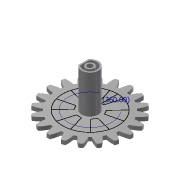
# Autodesk Inventor part: Spur Gear2
Saved by Autodesk Inventor 2018 (Build 220112000, 112)
## iProperties
Created: 2018-10-24
Part Number: Spur Gear2
Material: Steel
Document SubType Name: Modeling
Designer: Vulnic
Categories: <?xml version="1.0" encoding="UTF-16"?> <MemberInstance><Categories><FamilyTemplate><FamilyTemplateParameter ValueType="xs:double" Id="1" ObjectReferenceKey="da_z" ObjectType="kUserParameterObject"/><FamilyTemplateParameter ValueType="xs:double" Id="2" ObjectReferenceKey="da_b" ObjectType="kUserParameterObject"/><FamilyTemplateParameter ValueType="xs:double" Id="3" ObjectReferenceKey="da_beta" ObjectType="kUserParameterObject"/><FamilyTemplateParameter ValueType="xs:double" Id="4" ObjectReferenceKey="da_da" ObjectType="kUserParameterObject"/><FamilyTemplateParameter ValueType="xs:double" Id="5" ObjectReferenceKey="da_aw" ObjectType="kUserParameterObject"/><FamilyTemplateParameter ValueType="xs:string" Id="6" ObjectReferenceKey="EAIAABAAAACIAQAAAAAAAIAAAAAAAAAA" ObjectType="83910656" SubObjectId="SurfaceGeometry"/></FamilyTemplate><ParamToTemplateMap><ParamToTemplate CategoryParameter="//CategoryParameter[@InternalName='046C89C9-8512-4d59-83FE-43B91F4F132A']" TemplateParameter="1"/><ParamToTemplate CategoryParameter="//CategoryParameter[@InternalName='2552DF32-E462-4b46-AEBF-C6C7768E72AC']" TemplateParameter="2"/><ParamToTemplate CategoryParameter="//CategoryParameter[@InternalName='C9EE641D-15FC-4fae-A226-E94C4372FDD7']" TemplateParameter="3"/><ParamToTemplate><ParamToTemplate CategoryParameter="//CategoryParameter[@InternalName='00B6519A-459B-49c7-AD84-2E56D39A5744']" ConstantValue="0.000000"/></ParamToTemplate><ParamToTemplate><ParamToTemplate CategoryParameter="//CategoryParameter[@InternalName='04B31F0E-C7A6-4894-AA32-9629BEFACF47']" ConstantValue="1.000000"/></ParamToTemplate><ParamToTemplate><ParamToTemplate CategoryParameter="//CategoryParameter[@InternalName='43CBEC2E-7847-49e7-A936-2F7889FCB2D9']" ConstantValue="0.250000"/></ParamToTemplate><ParamToTemplate><ParamToTemplate CategoryParameter="//CategoryParameter[@InternalName='B1EFC894-105D-4ebd-86BF-FA20ED196853']" ConstantValue="0.350000"/></ParamToTemplate><ParamToTemplate><ParamToTemplate CategoryParameter="//CategoryParameter[@InternalName='51175063-3D10-4879-93E8-6246FE8B403D']" ConstantValue="2060000000.000000"/></ParamToTemplate><ParamToTemplate><ParamToTemplate CategoryParameter="//CategoryParameter[@InternalName='A3A52E27-4454-46a9-B0BD-C932399B70AF']" ConstantValue="0.300000"/></ParamToTemplate><ParamToTemplate><ParamToTemplate CategoryParameter="//CategoryParameter[@InternalName='91B76062-C214-41d9-B1B9-14D2AB99603D']" ConstantValue="0.100000"/></ParamToTemplate><ParamToTemplate><ParamToTemplate CategoryParameter="//CategoryParameter[@InternalName='374E806E-8B8A-4dda-A9AA-1039D6500AD2']" ConstantValue="10.000000"/></ParamToTemplate><ParamToTemplate><ParamToTemplate CategoryParameter="//CategoryParameter[@InternalName='2D373A89-B862-43d6-8D0B-0CBF12AB9F6C']" ConstantValue="0.349066"/></ParamToTemplate><ParamToTemplate CategoryParameter="//CategoryParameter[@InternalName='37777632-D6A2-4fac-9D53-DB8ACD95C989']" TemplateParameter="4"/><ParamToTemplate CategoryParameter="//CategoryParameter[@InternalName='FD1017F1-B727-4f7e-9707-0F86F1FF9423']" TemplateParameter="5"/><ParamToTemplate><ParamToTemplate CategoryParameter="//CategoryParameter[@InternalName='9E1B4470-B2D3-4ff1-B813-535BB4CDF51A']" ConstantValue="3520000.000000"/></ParamToTemplate><ParamToTemplate><ParamToTemplate CategoryParameter="//CategoryParameter[@InternalName='F8452263-BFF6-458c-9FB1-07C4B99E95CD']" ConstantValue="11400000.000000"/></ParamToTemplate><ParamToTemplate><ParamToTemplate CategoryParameter="//CategoryParameter[@InternalName='3E3BB259-FD49-497f-8171-6EBC954A3479']" ConstantValue="2.000000"/></ParamToTemplate><ParamToTemplate CategoryParameter="//CategoryParameter[@InternalName='27C3BAF2-7550-4e4b-AE2C-0DB134B7D9B7']" TemplateParameter="6"/></ParamToTemplateMap><Category DisplayName="Gear" InternalName="DC85795E-93AB-48d5-8EEE-5A27447B64BD" Mnemonic="Gear"><CategoryParameter DisplayName="z" InternalName="046C89C9-8512-4d59-83FE-43B91F4F132A" Mnemonic="z"/><CategoryParameter DisplayName="b" InternalName="2552DF32-E462-4b46-AEBF-C6C7768E72AC" Mnemonic="b"/><CategoryParameter DisplayName="||b|" InternalName="C9EE641D-15FC-4fae-A226-E94C4372FDD7" Mnemonic="beta"/><CategoryParameter DisplayName="x" InternalName="00B6519A-459B-49c7-AD84-2E56D39A5744" Mnemonic="x"/><CategoryParameter DisplayName="a*" InternalName="04B31F0E-C7A6-4894-AA32-9629BEFACF47" Mnemonic="a"/><CategoryParameter DisplayName="c*" InternalName="43CBEC2E-7847-49e7-A936-2F7889FCB2D9" Mnemonic="c"/><CategoryParameter DisplayName="r|.f|*" InternalName="B1EFC894-105D-4ebd-86BF-FA20ED196853" Mnemonic="rf"/><CategoryParameter DisplayName="E" InternalName="51175063-3D10-4879-93E8-6246FE8B403D" Mnemonic="E"/><CategoryParameter DisplayName="||m|" InternalName="A3A52E27-4454-46a9-B0BD-C932399B70AF" Mnemonic="mi"/><Category DisplayName="SpurGear" InternalName="26C5A22E-A91E-4dfd-A3B3-23CCAFAE1764" Mnemonic="SpurGear"><CategoryParameter DisplayName="m" InternalName="91B76062-C214-41d9-B1B9-14D2AB99603D" Mnemonic="m"/><CategoryParameter DisplayName="P" InternalName="374E806E-8B8A-4dda-A9AA-1039D6500AD2" Mnemonic="PP"/><CategoryParameter DisplayName="||a|" InternalName="2D373A89-B862-43d6-8D0B-0CBF12AB9F6C" Mnemonic="alpha"/><CategoryParameter DisplayName="d|.a|" InternalName="37777632-D6A2-4fac-9D53-DB8ACD95C989" Mnemonic="da"/><CategoryParameter DisplayName="a|.w|" InternalName="FD1017F1-B727-4f7e-9707-0F86F1FF9423" Mnemonic="aw"/><CategoryParameter DisplayName="||s||.Flim|" InternalName="9E1B4470-B2D3-4ff1-B813-535BB4CDF51A" Mnemonic="sFlim"/><CategoryParameter DisplayName="||s||.Hlim|" InternalName="F8452263-BFF6-458c-9FB1-07C4B99E95CD" Mnemonic="sHlim"/><CategoryParameter DisplayName="type" InternalName="3E3BB259-FD49-497f-8171-6EBC954A3479" Mnemonic="type"/><CategoryParameter DisplayName="PitchDiameter" InternalName="27C3BAF2-7550-4e4b-AE2C-0DB134B7D9B7" Mnemonic="IDS_PITCHDIAM"/></Category></Category></Categories></MemberInstance>
Density: 1 g/cm^3
Appearance: Steel
CustomPartVersion: 1
Author: Vulnic
Autodesk Inventor part; units mm, degrees
ref_plane "YZ Plane" through (0, 0, 0) normal (1, 0, 0) x (0, 1, 0)
ref_plane "XZ Plane" through (0, 0, 0) normal (0, 1, 0) x (-1, 0, 0)
ref_plane "XY Plane" through (0, 0, 0) normal (0, 0, 1) x (1, 0, 0)
sketch "Sketch1" plane through (0, 0, 0) normal (0, 0, 1) x (1, 0, 0)
  circle A0 centre (0, 0) radius 11
  dimension "d0" = 22
  constraints: 1 centre point
  measures "d0" diameter of A0
extrude "Extrusion1" add sketch "Sketch1" along normal blind 1
ref_plane "Work Plane2" through (0, 0, 0.5) normal (0, 0, 1) x (1, 0, 0)
sketch "Sketch2" plane through (0, 0, 0) normal (0, 0, -1) x (-1, 0, 0)
  circle A0 centre (0, 0) radius 11 projected
  circle A1 centre (0, 0) radius 10
  dimension "d3" = 20
  constraints: 1 centre point, 1 coincident
  measures "d3" diameter of A1
surface extrude "Pitch Diameter" sketch "Sketch2" against normal through all shown no curves A1
ref_plane "Work Plane8" through (0, 0, 0) normal (0.9876883, 0.1564345, 0) x (0, 0, 1)
ref_plane "Work Plane9" through (0, 0, 0) normal (1, 0, 0) x (0, 1, 0)
spur gear teeth "Spur Gear" teeth 20 pitch diameter 20 tip diameter 22 root diameter 17.5 face width 1 start plane through (0, 0, 0) normal (0, 0, -1) x (-1, 0, 0)
sketch "Sketch3" plane through (0, 0, 1) normal (0, 0, 1) x (1, 0, 0)
  circle A0 centre (0, 0) radius 2.2 projected
  line L0 (-1.7577, -1.323) -> (-1.7577, 1.323)
  point P0 (0, 0)
  dimension "d49" = 2.646
  constraints: 2 end point, 2 point on circle, 1 vertical
  measures "d49" distance of L0.start L0.end
extrude "Extrusion2" cut sketch "Sketch3" against normal through all contours A0 L0 picked at (-0.4385, 0)
sketch "Sketch4" plane through (0, 0, 1) normal (0, 0, 1) x (1, 0, 0)
  line L0 (-0.6517, 2.9374) -> (0.0047, 2.9374)
  line L1 (0.0047, 2.9374) -> (0.0047, 7.2274)
  circle A0 centre (0, 0) radius 7.2274
  line L2 (-0.6517, 2.9374) -> (-1.8312, 6.9916)
  line L3 (0.6611, 2.9374) -> (0.0047, 2.9374)
  line L4 (0.6611, 2.9374) -> (1.8406, 6.9916)
  line L5 (-2.2133, 2.0412) -> (-5.1346, 5.0898)
  line L6 (-2.2133, 2.0412) -> (-2.5415, 1.4727)
  line L7 (-2.8697, 0.9043) -> (-2.5415, 1.4727)
  line L8 (-2.8697, 0.9043) -> (-6.9705, 1.91)
  line L9 (-2.8744, -0.8961) -> (-6.9752, -1.9018)
  line L10 (-2.8744, -0.8961) -> (-2.5462, -1.4646)
  line L11 (-2.218, -2.0331) -> (-2.5462, -1.4646)
  line L12 (-2.218, -2.0331) -> (-5.1393, -5.0817)
  line L13 (-0.6611, -2.9374) -> (-1.8406, -6.9916)
  line L14 (-0.6611, -2.9374) -> (-0.0047, -2.9374)
  line L15 (0.6517, -2.9374) -> (-0.0047, -2.9374)
  line L16 (0.6517, -2.9374) -> (1.8312, -6.9916)
  line L17 (2.2133, -2.0412) -> (5.1346, -5.0898)
  line L18 (2.2133, -2.0412) -> (2.5415, -1.4727)
  line L19 (2.8697, -0.9043) -> (2.5415, -1.4727)
  line L20 (2.8697, -0.9043) -> (6.9705, -1.91)
  line L21 (2.8744, 0.8961) -> (6.9752, 1.9018)
  line L22 (2.8744, 0.8961) -> (2.5462, 1.4646)
  line L23 (2.218, 2.0331) -> (2.5462, 1.4646)
  line L24 (2.218, 2.0331) -> (5.1393, 5.0817)
  line L25 (0.6611, 2.9374) -> (0.0047, 2.9374)
  line L26 (0.6611, 2.9374) -> (1.8406, 6.9916)
  line L27 (2.8744, 0.8961) -> (2.218, 2.0331)
  line L28 (5.1393, 5.0817) -> (2.218, 2.0331)
  line L29 (2.8744, 0.8961) -> (7.0083, 1.91)
  line L30 (6.9705, -1.91) -> (2.9023, -0.9123)
  line L31 (2.2133, -2.0412) -> (5.133, -5.0881)
  line L32 (1.8312, -6.9916) -> (0.6517, -2.9374)
  line L33 (-0.6611, -2.9374) -> (0.6517, -2.9374)
  line L34 (-0.6611, -2.9374) -> (-1.8406, -6.9916)
  line L35 (2.2133, -2.0412) -> (2.8697, -0.9043)
  line L36 (2.2133, -2.0412) -> (5.133, -5.0881)
  line L37 (-2.218, -2.0331) -> (-2.8744, -0.8961)
  line L38 (-2.8744, -0.8961) -> (-6.9752, -1.9018)
  line L39 (-5.1393, -5.0817) -> (-2.218, -2.0331)
  line L40 (-6.9705, 1.91) -> (-2.8697, 0.9043)
  line L41 (-2.8697, 0.9043) -> (-2.2133, 2.0412)
  line L42 (-2.2133, 2.0412) -> (-5.1346, 5.0898)
  arc A1 (-6.9705, -1.91) -> (-5.1393, -5.0817) centre (0, 0) ccw
  dimension "d54" = 360
  constraints: 86 end point, 10 collinear, 6 point on circle, 3 point on line, 2 centre point, 2 parallel, 2 symmetric about line, 1 coincident, 1 concentric, 1 horizontal, 1 perpendicular, 55 other
shell "Shell1" thickness 0.4 removed faces 1 at (-4.0683, -0.3428, 0)
sketch "Sketch5" plane through (0, 0, 1) normal (0, 0, 1) x (1, 0, 0)
  arc A0 (-1.7577, -1.323) -> (-1.7577, 1.323) centre (0, 0) ccw projected
  line L0 (-1.7577, -1.323) -> (-1.7577, 1.323) projected
  point P0 (0, 0)
extrude "Extrusion3" add sketch "Sketch5" along normal blind 10
sketch "Sketch6" plane through (0, 0, 11) normal (0, 0, 1) x (1, 0, 0)
  circle A0 centre (0, 0) radius 0.7
  dimension "d59" = 1.4
  constraints: 1 centre point, 1 coincident
  measures "d59" diameter of A0
extrude "Extrusion4" cut sketch "Sketch6" against normal through all
sketch "Sketch7" plane through (0, 0, 1) normal (0, 0, -1) x (-1, 0, 0)
  line L0 (1.4807, 0.1822) -> (1.0807, 0.1822)
  line L1 (1.0807, 0.1822) -> (1.0807, -0.2178)
  line L2 (1.0807, -0.2178) -> (1.4807, -0.2178)
  line L3 (1.4807, -0.2178) -> (1.4807, 0.1822)
  line L4 (1.4807, 0.1822) -> (1.0807, -0.2178) construction
  line L5 (1.0807, 0.1822) -> (1.4807, -0.2178) construction
  line L6 (-0.3518, 1.0448) -> (-0.5518, 1.3912)
  line L7 (-0.8982, 1.1912) -> (-0.6982, 0.8448)
  line L8 (-0.6982, 0.8448) -> (-0.3518, 1.0448)
  line L9 (-0.5518, 1.3912) -> (-0.8982, 1.1912)
  line L10 (-0.7289, -0.827) -> (-0.9289, -1.1735)
  line L11 (-0.5825, -1.3735) -> (-0.3825, -1.027)
  line L12 (-0.3825, -1.027) -> (-0.7289, -0.827)
  line L13 (-0.9289, -1.1735) -> (-0.5825, -1.3735)
  point P0 (0, 0)
  point P1 (1.2807, -0.0178)
  dimension "d64" = 360
  dimension "d69" = 0.4
  constraints: 28 end point, 2 midpoint, 2 parallel, 2 perpendicular, 1 horizontal, 25 other
  measures "d69" distance of L0.end L1.end
extrude "Extrusion5" add sketch "Sketch7" along normal blind 1
shell "Shell2" thickness 0.4 removed faces 1 at (-1.4052, 0, 11)
equation "\"d0\" = da_da"
equation "\"d1\" = da_b"
equation "\"d3\" = da_dw"
equation "\"d16\" = da_aw"
equation "\"d43\" = da_aw"
equation "\"d46\" = da_aw"
equation "\"da_da\" = 22"
equation "\"da_b\" = 1"
equation "\"da_dw\" = 20"
equation "\"da_aw\" = 15"
body "Solid1"
body "Srf1"
